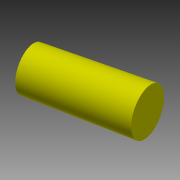
# Autodesk Inventor part: 32912_roller
Saved by Autodesk Inventor 2014 SP2 (Build 180246200, 246)
## iProperties
Created: 2018-11-12
Part Number: 32912_roller
Material: Generic
Catalog Web Link: www.cadenas.de
Description: BT1_001_101_roller-Tapered roller bearings, single row
Vendor: SKF
Document SubType Name: Modeling
Designer: psadmin
Manufacturer: SKF
Mass: 0.259208 g
Surface Area: 2.41857 cm^2
Volume: 0.259208 cm^3
Density: 1 g/cm^3
Appearance: PSOLRGB-255-255-0
Category: PARTsolutions
Company: SKF
Title: 32912_roller
Author: Cadenas PARTsolutions
Comments: Tapered roller bearings, single row
PSOL_IDENT_0: {$CADENAS_DATA\23d-libs\skf\bearings_units_and_housings\roller_bearings\tapered_roller_bearings\tape
PSOL_IDENT_1: red_roller_bearings_single_row\parts\bt1_001_101_roller.prj},178 {VTYP=3D},{NB=32912_roller},{LINA=3
PSOL_IDENT_2: 2912_roller},{NN=BT1_001_101_roller},{DATE=14.08.2018 07:35:10},{GEOMDATE=29.05.2018 10:30:25},{VERS
PSOL_IDENT_3: ION=},{LINEID=2140},{WBVAR=},{WBNUMERIC=}  {NB=32912_roller},{LINA=32912_roller},{KT=DUMMY},{DESIGNA
PSOL_IDENT_4: TION=32912},{DD=60.000},{D=85.000},{T=17.000},{DD1=73.8000},{D1=MIN},{B=17.000},{C=14.000},{C1=MIN},
PSOL_IDENT_5: {R12=1.0},{R34=1.0},{AA=15.45165},{PITCH=72.347},{DW=5.200},{LW=12.200},{RANGLE=1.600},{ALPHA=12.450
PSOL_IDENT_6: },{DDAMAX=67},{DDAMIN=68.0},{DAMIN=78},{DAMAX=78.0},{DBMIN=81},{CA=3},{CB=3.0},{RA=1.0},{RB=1.0},{LO
PSOL_IDENT_7: AD1=53.200},{LOAD2=75.000},{LOAD3=7.800},{SPEED1=6000},{SPEED2=7000},{EE=0.33},{Y=1.80},{Y0=1.0},{Y1=
PSOL_IDENT_8: 0},{X1=1},{X2=0.4},{X0=0.5},{Z=34},{II=1},{R1=0.00000231},{R2=10.9},{S1=0.009},{S2=2},{KZ=6},{KL=0.7
PSOL_IDENT_9: },{BF=2},{MASS=0.302},{PIM=PIM_BT1_001},{DESIGN=trb1},{HELP=0.000}
NN: BT1_001_101_roller
NT: Tapered roller bearings, single row
NB: 32912_roller
NBSYN: $DESIGNATION._roller
LINA: 32912_roller
DESIGNATION: 32912
DD: 60
D: 85
T: 17
DD1: 73.8
D1: 0
B: 17
C: 14
C1: 0
R12: 1
R34: 1
AA: 15.45165
PITCH: 72.347
DW: 5.2
LW: 12.2
RANGLE: 1.6
ALPHA: 12.45
DDAMAX: 67
DDAMIN: 68
DAMIN: 78
DAMAX: 78
DBMIN: 81
CA: 3
CB: 3
RA: 1
RB: 1
LOAD1: 53.2
LOAD2: 75
LOAD3: 7.8
SPEED1: 6000
SPEED2: 7000
EE: 0.33
Y: 1.8
Y0: 1
Y1: 0
X1: 1
X2: 0.4
X0: 0.5
Z: 34
II: 1
R1: 0.00000231
R2: 10.9
S1: 0.009
S2: 2
KZ: 6
KL: 0.7
BF: 2
MASS: 0.302
PIM: PIM_BT1_001
SUPPLIER: SKF
ARTICLENO: 32912_roller
BOMINFO: 32912_roller
CREATOR: CADENAS GmbH
Autodesk Inventor part; units mm, degrees
sketch "Sketch_1" plane through (0, 0, 0) normal (0, 0, 1) x (1, 0, 0)
  line L0 (13.4218, 37.4886) -> (1.5087, 34.8584)
  line L1 (1.5087, 34.8584) -> (0.9686, 37.305)
  line L2 (0.9686, 37.305) -> (12.8409, 40.1197)
  line L3 (12.8409, 40.1197) -> (13.4218, 37.4886)
  line L4 (13.4218, 37.4886) -> (1.5087, 34.8584)
  constraints: 10 end point
revolve "Revolution1" add sketch "Sketch_1" angle 360 about axis through (13.4218, 37.4886, 0) along (0.9764845, 0.2155876, 0)
ref_plane "roller_XY" through (0, 36.1735, 0) normal (-1, 0, 0) x (0, 0, -1)
ref_plane "roller_YZ" through (0, 36.1735, 0) normal (0, 0, -1) x (0, -1, 0)
ref_plane "roller_ZX" through (0, 36.1735, 0) normal (0, -1, 0) x (-1, 0, 0)
body "Solid1"
